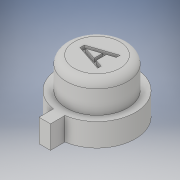
# Autodesk Inventor part: ButtonA_neu
Saved by Autodesk Inventor 2019 (Build 230136000, 136)
## iProperties
Created: 2020-09-24
Part Number: ButtonA_neu
Material: Generisch
Document SubType Name: Modeling
Designer: David
Density: 1 g/cm^3
Appearance: Vorgabe
Author: David
Autodesk Inventor part; units mm, degrees
ref_plane "YZ Plane" through (0, 0, 0) normal (1, 0, 0) x (0, 1, 0)
ref_plane "XZ Plane" through (0, 0, 0) normal (0, 1, 0) x (-1, 0, 0)
ref_plane "XY Plane" through (0, 0, 0) normal (0, 0, 1) x (1, 0, 0)
sketch "Skizze1" plane through (0, 0, 0) normal (1, 0, 0) x (0, 1, 0)
  line L0 (4, 0) -> (4, 3)
  arc A0 (4, 3) -> (3, 4) centre (3, 3) ccw
  line L1 (3, 4) -> (0, 4)
  line L2 (0, 4) -> (0, 5)
  line L3 (0, 5) -> (-3, 5)
  line L4 (-3, 5) -> (-3, 2)
  line L5 (0, 0) -> (4, 0)
  line L6 (-3, 2) -> (-3, 0)
  line L7 (-3, 0) -> (0, 0)
  point P0 (0, 2)
  dimension "d0" = 2
  dimension "d1" = 4
  dimension "d2" = 3
  dimension "d3" = 5
  dimension "d4" = 3
  dimension "d5" = 1
  dimension "d6" = 1
  constraints: 16 end point, 4 perpendicular, 2 point on circle, 2 vertical, 1 centre point, 1 horizontal, 1 point on line, 1 tangent
  measures "d0" distance of point (0, 2) L5.start
  measures "d1" distance between parallel lines of L5 L1
  measures "d2" distance of L4.end point (0, 2)
  measures "d3" distance between parallel lines of L5 L3
  measures "d4" distance of L1.start L1.end
  measures "d5" distance from line of L1.start L0
  measures "d6" horizontal distance of L1.start L0.end
revolve "Umdrehung1" add sketch "Skizze1" angle 360 about axis through (0, 0, 0) along (0, 1, 0)
sketch "Skizze2" plane through (0, 4, 0) normal (0, 1, 0) x (1, 0, 0)
  line L0 (-1.9622, -1.4344) -> (-1.9622, 1.4984) construction
  line L1 (-1.9622, 1.4984) -> (1.5378, 1.4984) construction
  line L2 (1.5378, 1.4984) -> (1.5378, -1.4344) construction
  line L3 (1.5378, -1.4344) -> (-1.9622, -1.4344) construction
  line L4 (1.5378, -1.457) -> (-1.9622, -0.2771)
  line L5 (-1.9622, -0.2771) -> (-1.9622, 0.2958)
  line L6 (-1.9622, 0.2958) -> (1.5378, 1.4757)
  line L7 (1.5378, 1.4757) -> (1.5378, 0.985)
  line L8 (1.5378, 0.985) -> (0.5593, 0.6673)
  line L9 (0.5593, 0.6673) -> (0.5593, -0.6686)
  line L10 (0.5593, -0.6686) -> (1.5378, -0.9862)
  line L11 (1.5378, -0.9862) -> (1.5378, -1.457)
  line L12 (0.1622, 0.5397) -> (-1.4857, -0.002)
  line L13 (-1.4857, -0.002) -> (0.1622, -0.5409)
  line L14 (0.1622, -0.5409) -> (0.1622, 0.5397)
  point P0 (0, 0)
  constraints: 2 other
extrude "Extrusion1" cut sketch "Skizze2" against normal blind 0.5
sketch "Skizze4" plane through (0, -3, 0) normal (0, -1, 0) x (1, 0, 0)
  line L0 (0.75, 6.8364) -> (-0.75, 6.8364)
  line L1 (-0.75, 6.8364) -> (-0.75, 4.8364)
  line L2 (-0.75, 4.8364) -> (0.75, 4.8364)
  line L3 (0.75, 4.8364) -> (0.75, 6.8364)
  point P0 (0, 0)
  dimension "d15" = 1.5
  dimension "d16" = 2
  dimension "d19" = 0.75
  constraints: 8 end point, 2 parallel, 1 horizontal, 1 perpendicular
  measures "d15" distance of L1.end L2.end
  measures "d16" distance between parallel lines of L2 L0
  measures "d19" distance from line of point (0, 0) L1
extrude "Extrusion3" add sketch "Skizze4" against normal blind 3
